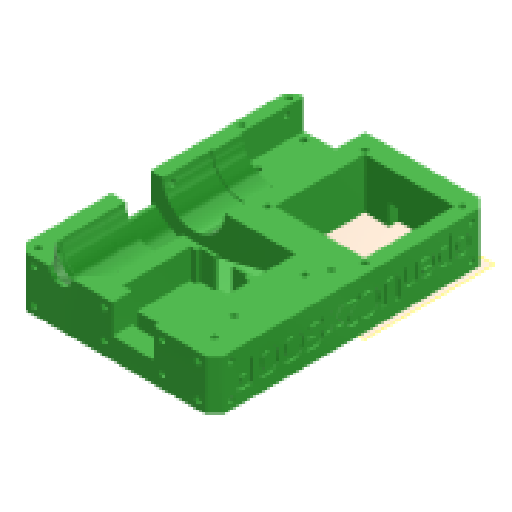
# Autodesk Inventor part: 60_Planktoscope_Base_half1
Saved by Autodesk Inventor 2024.1 (Build 281209000, 209)
## iProperties
Created: 2024-03-03
Part Number: 60_Planktoscope_Base_half1
Material: Generisch
Document SubType Name: Modeling
Designer: diederichbenedict
Density: 1 g/cm^3
Appearance: Glatt - Waldgrün
Author: diederichbenedict
Autodesk Inventor part; units mm, degrees
(part 1 of 2)
ref_plane "YZ Plane" through (0, 0, 0) normal (1, 0, 0) x (0, 1, 0)
ref_plane "XZ Plane" through (0, 0, 0) normal (0, 1, 0) x (-1, 0, 0)
ref_plane "XY Plane" through (0, 0, 0) normal (0, 0, 1) x (1, 0, 0)
ref_plane "Arbeitsebene1" through (0, 0, 0) normal (0, 0, 1) x (1, 0, 0)
ref_plane "Arbeitsebene2" through (-59.4, -108.46, 24.3) normal (0, 0, -1) x (0, 1, 0)
sketch "Skizze1" plane through (0, 0, 0) normal (0, 0, 1) x (1, 0, 0)
  line L0 (-24.5, 28.5) -> (24.5, 28.5) construction
  arc A0 (-24.5, 28.5) -> (-28.5, 24.5) centre (-24.5, 24.5) ccw construction
  line L1 (-28.5, -24.5) -> (-28.5, 24.5) construction
  arc A1 (-28.5, -24.5) -> (-24.5, -28.5) centre (-24.5, -24.5) ccw construction
  line L2 (24.5, -28.5) -> (-24.5, -28.5) construction
  arc A2 (24.5, -28.5) -> (28.5, -24.5) centre (24.5, -24.5) ccw construction
  line L3 (28.5, 24.5) -> (28.5, -24.5) construction
  arc A3 (28.5, 24.5) -> (24.5, 28.5) centre (24.5, 24.5) ccw construction
  circle A4 centre (15.5, -15.5) radius 2 construction
  circle A5 centre (-15.5, -15.5) radius 2 construction
  circle A6 centre (-15.5, 15.5) radius 2 construction
  circle A7 centre (15.5, 15.5) radius 2 construction
  circle A8 centre (0, 0) radius 11.5 construction
  circle A9 centre (23.5, -23.5) radius 2 construction
  circle A10 centre (-23.5, -23.5) radius 2 construction
  circle A11 centre (-23.5, 23.5) radius 2 construction
  circle A12 centre (23.5, 23.5) radius 2 construction
  line L4 (21.15, 14.15) -> (21.15, -14.15) construction
  line L5 (14.15, 21.15) -> (21.15, 14.15) construction
  line L6 (-14.15, 21.15) -> (14.15, 21.15) construction
  line L7 (-21.15, 14.15) -> (-14.15, 21.15) construction
  line L8 (-21.15, -14.15) -> (-21.15, 14.15) construction
  line L9 (-14.15, -21.15) -> (-21.15, -14.15) construction
  line L10 (14.15, -21.15) -> (-14.15, -21.15) construction
  line L11 (21.15, -14.15) -> (14.15, -21.15) construction
  line L12 (17.15, 21.15) -> (14.15, 21.15) construction
  line L13 (21.15, 14.15) -> (14.15, 21.15) construction
  line L14 (21.15, 14.15) -> (21.15, 17.15) construction
  line L15 (21.15, 17.15) -> (17.15, 21.15) construction
  line L16 (21.1433, 21.15) -> (-21.15, 21.15) construction
  line L17 (-21.15, 21.15) -> (-21.15, -21.15) construction
  line L18 (-21.15, -21.15) -> (21.1433, -21.15) construction
  line L19 (21.1433, -21.15) -> (21.1433, 21.15) construction
  line L20 (21.6433, 21.65) -> (-21.65, 21.65)
  line L21 (-21.65, 21.65) -> (-21.65, -21.65)
  line L22 (-21.65, -21.65) -> (21.6433, -21.65)
  line L23 (21.6433, -21.65) -> (21.6433, 21.65)
  circle A13 centre (23.5, 23.5) radius 1.4
  circle A14 centre (23.5, -23.5) radius 1.4
  circle A15 centre (-23.5, 23.5) radius 1.4
  circle A16 centre (-23.5, -23.5) radius 1.4
  line L24 (-58.0629, 31.15) -> (-46.7147, 31.15) construction
  line L25 (-24.5, 28.5) -> (24.5, 28.5) construction
  line L26 (-58.15, -108.944) -> (-33.15, -108.944) construction
  line L27 (-60.15, 4.6456) -> (-60.15, 29.65) construction
  line L28 (28.5, 31.15) -> (-66.5, 31.15) construction
  line L29 (-66.5, 31.15) -> (-66.5, -100.85) construction
  line L30 (-66.5, -100.85) -> (28.5, -100.85) construction
  line L31 (28.5, -100.85) -> (28.5, 31.15) construction
  line L32 (28.5, 31.15) -> (-66.5, 31.15)
  line L33 (-66.5, 31.15) -> (-66.5, -100.85)
  line L34 (-66.5, -100.85) -> (28.5, -100.85)
  line L35 (28.5, -100.85) -> (28.5, 31.15)
  circle A17 centre (-34.65, 27.15) radius 1.6 projected
  circle A18 centre (-35.65, 4.15) radius 1.55 projected
  arc A19 (-35.0696, 29.65) -> (-37.5716, 27.1718) centre (-35.0717, 27.15) ccw construction
  line L36 (-32.3578, 29.6503) -> (-35.0696, 29.6501) construction
  line L37 (-32.3578, 29.6503) -> (-32.3574, 2.149) construction
  spline S0 degree 3 poles (-33.2494, 1.4648) (-33.1945, 1.4704) (-33.1402, 1.4798) (-33.0852, 1.4932) (-33.0302, 1.5066) (-32.9745, 1.5241) (-32.9218, 1.5443) (-32.869, 1.5646) (-32.8192, 1.5877) (-32.7741, 1.6117) (-32.729, 1.6358) (-32.6887, 1.6608) (-32.6523, 1.6864) (-32.6158, 1.712) (-32.5833, 1.7382) (-32.5542, 1.7648) (-32.5251, 1.7914) (-32.4996, 1.8183) (-32.4775, 1.8453) (-32.4554, 1.8722) (-32.4367, 1.899) (-32.4213, 1.9255) (-32.4059, 1.952) (-32.3937, 1.978) (-32.3842, 2.0033) (-32.3747, 2.0286) (-32.3679, 2.0532) (-32.3636, 2.0778) (-32.3593, 2.1023) (-32.3574, 2.1268) (-32.3574, 2.149) knots 0 0 0 0 0.1 0.1 0.1 0.2 0.2 0.2 0.3 0.3 0.3 0.4 0.4 0.4 0.5 0.5 0.5 0.6 0.6 0.6 0.7 0.7 0.7 0.8 0.8 0.8 0.9 0.9 0.9 1 1 1 1 construction
  spline S1 degree 3 poles (-58.0506, 1.4648) (-57.9483, 1.4544) (-57.7309, 1.4485) (-57.3891, 1.4505) (-57.0142, 1.4499) (-56.6055, 1.45) (-56.1597, 1.45) (-55.6728, 1.45) (-55.1399, 1.45) (-54.5557, 1.45) (-53.9136, 1.45) (-53.2059, 1.45) (-52.4235, 1.45) (-51.5547, 1.45) (-50.5859, 1.45) (-49.498, 1.45) (-48.2725, 1.45) (-46.9373, 1.45) (-45.5731, 1.45) (-44.2623, 1.45) (-43.0442, 1.45) (-41.9119, 1.45) (-40.8595, 1.45) (-39.8813, 1.45) (-38.9722, 1.45) (-38.1274, 1.45) (-37.3425, 1.45) (-36.6135, 1.45) (-35.9369, 1.45) (-35.3097, 1.45) (-34.7295, 1.45) (-34.1949, 1.45) (-33.7068, 1.4499) (-33.3956, 1.4501) (-33.2494, 1.4648) knots 0 0 0 0 0.012454 0.026265 0.041356 0.057789 0.075708 0.095278 0.116688 0.140158 0.165945 0.194355 0.225757 0.26059 0.299437 0.342945 0.392182 0.44767 0.504448 0.55719 0.606219 0.651791 0.694148 0.733518 0.770107 0.804111 0.835704 0.865049 0.892289 0.917546 0.940917 0.962464 0.982201 1 1 1 1 construction
  spline S2 degree 3 poles (-58.9429, 2.1479) (-58.9428, 2.1323) (-58.9408, 2.1003) (-58.9319, 2.0518) (-58.9165, 2.0024) (-58.8947, 1.9528) (-58.866, 1.9029) (-58.8299, 1.8528) (-58.786, 1.8026) (-58.7333, 1.7522) (-58.6711, 1.7019) (-58.5978, 1.6519) (-58.512, 1.6028) (-58.4118, 1.556) (-58.2981, 1.5143) (-58.1761, 1.4822) (-58.092, 1.469) (-58.0506, 1.4648) knots 0.000644 0.000644 0.000644 0.000644 0.046478 0.094952 0.144249 0.194804 0.247064 0.301535 0.358802 0.419552 0.484614 0.554981 0.631878 0.716385 0.809647 0.906987 1 1 1 1 construction
  line L38 (-58.9426, 2.1485) -> (-58.9422, 29.6503) construction
  line L39 (-58.9422, 29.6503) -> (-56.2298, 29.6501) construction
  arc A20 (-53.7284, 27.1718) -> (-56.2298, 29.65) centre (-56.2283, 27.15) ccw construction
  line L40 (-53.7228, 26.5387) -> (-53.7284, 27.1718) construction
  arc A21 (-53.7228, 26.5387) -> (-52.4229, 25.25) centre (-52.4229, 26.55) ccw construction
  line L41 (-38.8771, 25.25) -> (-52.4229, 25.25) construction
  arc A22 (-38.8771, 25.25) -> (-37.5772, 26.5387) centre (-38.8771, 26.55) ccw construction
  line L42 (-37.5772, 26.5387) -> (-37.5716, 27.1718) construction
  circle A23 centre (-56.65, 27.15) radius 1.6 projected
  line L43 (-58.35, 24.2) -> (-35.55, 24.2) construction
  line L44 (-58.35, 8.8) -> (-58.35, 24.2) construction
  line L45 (-32.95, 8.8) -> (-58.35, 8.8) construction
  line L46 (-32.95, 21.2) -> (-32.95, 8.8) construction
  line L47 (-35.55, 24.2) -> (-32.95, 21.2) construction
  circle A24 centre (-55.65, 4.15) radius 1.55 projected
  circle A25 centre (-51.65, 5.65) radius 1.1 construction
  circle A26 centre (-39.65, 5.65) radius 1.1 construction
  circle A27 centre (-35.65, 4.15) radius 1.55 construction
  circle A28 centre (-34.65, 27.15) radius 1.6 construction
  point P0 (0, 0)
  dimension "d0" = 0.5
  dimension "d1" = 2.8
  dimension "d2" = 2.8
  dimension "d3" = 2.8
  dimension "d4" = 2.8
  dimension "d5" = 95
  dimension "d6" = 132
  dimension "d41" = 31.15
  constraints: 32 end point, 8 parallel, 4 centre point, 4 coincident, 4 perpendicular, 3 horizontal, 3 other
  measures "d0" distance between parallel lines of L19 L23
  measures "d1" diameter of A13
  measures "d2" diameter of A14
  measures "d3" diameter of A15
  measures "d4" diameter of A16
  measures "d5" distance of L30.end L29.end
  measures "d6" distance of L29.end L28.end
  measures "d41" distance from line of L28 point (0, 0)
extrude "Extrusion1" add sketch "Skizze1" along normal up to surface (24.3 mm away)
sketch "Skizze2" plane through (-66.5, 31.15, 24.3) normal (0, 0, 1) x (1, 0, 0)
  line L0 (44.85, -9.5) -> (88.1433, -9.5) projected
  line L1 (88.1433, -9.5) -> (88.1433, -52.8) projected
  line L2 (88.1433, -52.8) -> (44.85, -52.8) projected
  line L3 (44.85, -52.8) -> (44.85, -9.5) projected
  circle A0 centre (90, -7.65) radius 1.4 projected
  circle A1 centre (90, -54.65) radius 1.4 projected
  circle A2 centre (43, -7.65) radius 1.4 projected
  circle A3 centre (43, -54.65) radius 1.4 projected
  circle A4 centre (31.85, -4) radius 1.6 projected
  circle A5 centre (30.85, -27) radius 1.55 projected
  circle A6 centre (9.85, -4) radius 1.6 projected
  circle A7 centre (10.85, -27) radius 1.55 projected
  line L4 (95, 0) -> (0, 0) projected
  line L5 (0, 0) -> (0, -132) projected
  line L6 (0, -132) -> (95, -132) projected
  line L7 (95, -132) -> (95, 0) projected
  line L8 (7.35, -118.91) -> (7.35, -120.06)
  arc A8 (7.35, -118.91) -> (7.35, -117.91) centre (7.35, -118.41) ccw construction
  line L9 (7.35, -96.06) -> (7.35, -117.91) construction
  line L10 (7.35, -85.56) -> (7.35, -94.56)
  line L11 (6.25, -85.56) -> (35.45, -85.56) projected
  line L12 (6.25, -70.56) -> (6.25, -85.56)
  line L13 (6.25, -44.56) -> (6.25, -70.06)
  line L14 (6.9535, -41.86) -> (6.8517, -30.1979)
  line L15 (33.2, -30.2) -> (33.2, -41.66)
  line L16 (6.9, -41.86) -> (6.9, -44.56)
  line L17 (6.25, -44.56) -> (35.45, -44.56) projected
  line L18 (20.85, -132) -> (20.85, 0) construction
  line L19 (15.35, -128.06) -> (15.35, -132)
  line L20 (7.35, -96.06) -> (7.35, -94.56)
  line L21 (7.35, -85.56) -> (6.25, -85.56)
  line L22 (6.25, -70.56) -> (6.25, -70.06)
  line L23 (15.1, -132) -> (15.1, -128.1636)
  line L24 (7.1, -120.1636) -> (7.1, -118.41)
  arc A9 (7.1, -118.41) -> (7.1, -118.41) centre (7.35, -118.41) ccw
  line L25 (7.1, -118.41) -> (7.1, -96.0507)
  line L26 (7.1, -96.0507) -> (7.1, -94.56)
  line L27 (7.1, -94.56) -> (7.1, -85.81)
  line L28 (7.1, -85.81) -> (6, -85.81)
  line L29 (6, -85.81) -> (6, -70.56)
  line L30 (6, -70.56) -> (6, -70.06)
  line L31 (6, -70.06) -> (6, -44.31)
  line L32 (6, -44.31) -> (35.45, -44.31)
  line L33 (6.8, -44.31) -> (6.8, -30.064)
  line L34 (6.8, -30.064) -> (20.85, -30.064)
  line L35 (20.85, -30.064) -> (20.85, -132)
  line L36 (15.1, -132) -> (20.85, -132)
  line L37 (7.1, -97.4127) -> (7.2407, -96.0654)
  line L38 (7.2407, -96.0654) -> (7.1, -96.0507)
  circle A10 centre (7.1, -117.9136) radius 0.5
  line L39 (7.35, -120.06) -> (15.35, -129.594) construction
  line L40 (15.35, -130.03) -> (7.1, -120.198)
  line L41 (7.1, -120.198) -> (7.1, -120.1636)
  point P0 (66.5, -31.15)
  point P1 (20.85, -85.56)
  point P2 (20.85, -44.56)
  point P3 (20.85, -44.31)
  point P4 (7.1, -118.4136)
  point P5 (7.1, -117.4136)
  point P6 (15.1, -129.7321)
  point P7 (6.9, -44.31)
  dimension "d9" = 0.25
  dimension "d74" = 1
  dimension "d75" = 2.25
  constraints: 64 end point, 11 vertical, 7 point on line, 5 perpendicular, 4 point on circle, 3 centre point, 2 collinear, 1 horizontal, 1 midpoint, 1 parallel, 30 other
  measures "d9" distance between parallel lines of L9 L25
  measures "d74" diameter of A10
  measures "d75" distance of A10.centre L24.start
revolve "Umdrehung1" cut sketch "Skizze2" angle 360 about axis through (-45.65, -100.85, 24.3) along (0, 1, 0) contours L6 L19 L40 L41 L24 A9 A10 L25 L37 L38 L26 L27 L28 L29 L30 L31 L32 L16 L17 L13 L22 L12 L11 L35 | L11 L12 L22 L13 L17 L35 | L17 L16 L32 L35 | L32 L33 L34 L35 | A10 A9
sketch "Skizze3" plane through (-66.5, 31.15, 24.3) normal (0, 0, 1) x (1, 0, 0)
  line L0 (41.8499, -119.66) -> (41.8499, -113.96) projected
  line L1 (69.8499, -119.66) -> (69.8499, -113.96) projected
  line L2 (47.9499, -122.06) -> (63.7499, -122.06) projected
  line L3 (44.8499, -88.76) -> (66.8499, -88.76) projected
  line L4 (44.8499, -90.56) -> (44.8499, -88.76)
  line L5 (66.8499, -90.56) -> (66.8499, -88.76)
  line L6 (41.8499, -122.06) -> (69.8499, -122.06)
  line L7 (69.8499, -122.06) -> (69.8499, -90.56)
  line L8 (69.8499, -90.56) -> (41.8499, -90.56)
  line L9 (41.8499, -90.56) -> (41.8499, -122.06)
  line L10 (65.8499, -140.6578) -> (45.8499, -140.6578)
  line L11 (45.8499, -140.6578) -> (45.8499, -122.06)
  line L12 (45.8499, -122.06) -> (65.8499, -122.06)
  line L13 (65.8499, -122.06) -> (65.8499, -140.6578)
  line L14 (65.8499, -140.6578) -> (45.8499, -122.06) construction
  line L15 (45.8499, -140.6578) -> (65.8499, -122.06) construction
  line L16 (41.3499, -122.56) -> (70.3499, -122.56)
  line L17 (70.3499, -122.56) -> (70.3499, -90.06)
  line L18 (70.3499, -90.06) -> (41.3499, -90.06)
  line L19 (41.3499, -90.06) -> (41.3499, -122.56)
  line L20 (67.3499, -90.56) -> (67.3499, -88.26)
  line L21 (67.3499, -88.26) -> (44.3499, -88.26)
  line L22 (44.3499, -88.26) -> (44.3499, -90.56)
  line L23 (60.0306, -74.6503) -> (51.6692, -74.6503)
  line L24 (51.6692, -74.6503) -> (51.6692, -88.26)
  line L25 (51.6692, -88.26) -> (60.0306, -88.26)
  line L26 (60.0306, -88.26) -> (60.0306, -74.6503)
  line L27 (60.0306, -74.6503) -> (51.6692, -88.26) construction
  line L28 (51.6692, -74.6503) -> (60.0306, -88.26) construction
  point P0 (66.5, -31.15)
  point P1 (55.8499, -131.3589)
  point P2 (55.8499, -81.4552)
  point P3 (44.3499, -90.06)
  point P4 (45.8499, -122.56)
  point P5 (65.8499, -122.56)
  point P6 (67.3499, -90.06)
  dimension "d11" = 20
  dimension "d12" = 0.5
  dimension "d13" = 0.5
  constraints: 50 end point, 8 parallel, 4 midpoint, 4 perpendicular, 3 horizontal, 2 point on line, 2 vertical, 7 other
  measures "d11" distance of L11.end L12.end
  measures "d12" distance between parallel lines of L9 L19
  measures "d13" distance between parallel lines of L3 L21
extrude "Extrusion2" cut sketch "Skizze3" against normal blind 14.1
sketch "Skizze4" plane through (-60.5, -54.66, 24.3) normal (0, 1, 0) x (1, 0, 0)
  arc A0 (14.7163, 14.1976) -> (0.6736, 0.7871) centre (14.85, 0) ccw projected
  circle A1 centre (49.8499, -0.1) radius 2.3 projected
  circle A2 centre (14.85, 0) radius 14.1983
  circle A3 centre (49.8499, -0.1) radius 6
  circle A4 centre (14.85, 0) radius 22.1983
  circle A5 centre (49.8499, -0.1) radius 14
  line L0 (20.1113, 21.5658) -> (53.168, 13.5011)
  line L1 (49.8499, -0.1) -> (14.85, 0)
  point P0 (60.5, 24.3)
  point P1 (37.0482, -0.0634)
  point P2 (35.8499, -0.06)
  point P3 (36.5766, -4.5519)
  point P4 (36.6022, 4.4277)
  dimension "d16" = 12
  dimension "d17" = 8
  dimension "d18" = 8
  constraints: 4 end point, 2 centre point, 2 coincident, 1 concentric, 8 other
  measures "d16" diameter of A3
extrude "Extrusion3" cut sketch "Skizze4" along normal blind 18 and the other way blind 1 contours A2 A0 | A1 | A3 | A4 L1 A5 | A4 A5 | A5 A4 | A4 L0 A5 | A4 A5 L1
sketch "Skizze5" plane through (-66.5, 31.15, 24.3) normal (0, 0, 1) x (1, 0, 0)
  line L0 (60.0306, -86.81) -> (60.0306, -88.26) projected
  line L1 (60.0306, -88.26) -> (67.3499, -88.26) projected
  line L2 (67.3499, -88.26) -> (67.3499, -90.06) projected
  line L3 (67.3499, -90.06) -> (70.3499, -90.06) projected
  line L4 (70.3499, -90.06) -> (70.3499, -122.56) projected
  line L5 (70.3499, -122.56) -> (65.8499, -122.56) projected
  line L6 (65.8499, -122.56) -> (65.8499, -132) projected
  line L7 (65.8499, -132) -> (95, -132) projected
  line L8 (95, -132) -> (95, 0) projected
  line L9 (95, 0) -> (0, 0) projected
  line L10 (26.35, -132) -> (45.8499, -132) projected
  line L11 (44.85, -9.5) -> (88.1433, -9.5) projected
  line L12 (88.1433, -9.5) -> (88.1433, -52.8) projected
  line L13 (88.1433, -52.8) -> (44.85, -52.8) projected
  line L14 (44.85, -52.8) -> (44.85, -9.5) projected
  circle A0 centre (90, -7.65) radius 1.4 projected
  circle A1 centre (90, -54.65) radius 1.4 projected
  circle A2 centre (43, -7.65) radius 1.4 projected
  circle A3 centre (43, -54.65) radius 1.4 projected
  circle A4 centre (31.85, -4) radius 1.6 projected
  circle A5 centre (30.85, -27) radius 1.55 projected
  circle A6 centre (9.85, -4) radius 1.6 projected
  circle A7 centre (10.85, -27) radius 1.55 projected
  line L15 (35.35, -1.5) -> (35.35, -27) projected
  line L16 (6.35, -26.9997) -> (6.35, -1.5) projected
  line L17 (35.35, -30.064) -> (6.35, -30.064)
  line L18 (6.35, -30.064) -> (6.35, 0)
  line L19 (6.35, 0) -> (35.35, 0)
  line L20 (35.35, 0) -> (35.35, -30.064)
  line L21 (35.65, -30.364) -> (6.05, -30.364)
  line L22 (6.05, -30.364) -> (6.05, 0.3)
  line L23 (6.05, 0.3) -> (35.65, 0.3)
  line L24 (35.65, 0.3) -> (35.65, -30.364)
  line L25 (45.8499, -132) -> (45.8499, -122.56) projected
  line L26 (45.8499, -122.56) -> (41.3499, -122.56) projected
  line L27 (41.3499, -122.56) -> (41.3499, -90.06) projected
  line L28 (41.3499, -90.06) -> (44.3499, -90.06) projected
  line L29 (44.3499, -90.06) -> (44.3499, -88.26) projected
  line L30 (44.3499, -88.26) -> (51.6692, -88.26) projected
  line L31 (51.6692, -88.26) -> (51.6692, -86.81) projected
  line L32 (0, -86.81) -> (0, -132) projected
  line L33 (51.6692, -86.81) -> (34.6, -86.81) projected
  line L34 (34.6, -86.81) -> (34.6, -96.0507) projected
  line L35 (34.6, -96.0507) -> (34.4593, -96.0654) projected
  line L36 (34.4593, -96.0654) -> (34.6, -97.4127) projected
  line L37 (34.6, -97.4127) -> (34.6, -117.4136) projected
  arc A8 (34.6, -117.4136) -> (34.6, -118.4136) centre (34.6, -117.9136) ccw projected
  line L38 (34.6, -118.4136) -> (34.6, -120.198) projected
  line L39 (34.6, -120.198) -> (26.35, -130.03) projected
  line L40 (26.35, -130.03) -> (26.35, -132) projected
  line L41 (69.8495, -86.81) -> (60.0306, -86.81) projected
  line L42 (0, 0) -> (0, -67.81) projected
  line L43 (0, -67.81) -> (6, -67.81) projected
  line L44 (6, -67.81) -> (6, -44.31) projected
  line L45 (6, -44.31) -> (6.8, -44.31) projected
  line L46 (6.8, -44.31) -> (6.8, -30.064) projected
  line L47 (6.8, -30.064) -> (34.9, -30.064) projected
  line L48 (34.9, -30.064) -> (34.9, -44.31) projected
  line L49 (34.9, -44.31) -> (35.7, -44.31) projected
  line L50 (35.7, -44.31) -> (35.7, -67.81) projected
  line L51 (35.7, -67.81) -> (69.8495, -67.81) projected
  line L52 (69.8495, -67.81) -> (69.8495, -86.81) projected
  line L53 (7.1, -86.81) -> (0, -86.81) projected
  line L54 (0, -132) -> (15.35, -132) projected
  line L55 (15.35, -132) -> (15.35, -130.03) projected
  line L56 (15.35, -130.03) -> (7.1, -120.198) projected
  line L57 (7.1, -120.198) -> (7.1, -118.4136) projected
  arc A9 (7.1, -118.4136) -> (7.1, -117.4136) centre (7.1, -117.9136) ccw projected
  line L58 (7.1, -117.4136) -> (7.1, -97.4127) projected
  line L59 (7.1, -97.4127) -> (7.2407, -96.0654) projected
  line L60 (7.2407, -96.0654) -> (7.1, -96.0507) projected
  line L61 (7.1, -96.0507) -> (7.1, -86.81) projected
  point P0 (66.5, -31.15)
  dimension "d23" = 0.3
  constraints: 16 end point, 4 parallel, 2 perpendicular, 1 horizontal, 1 point on line, 3 other
  measures "d23" distance between parallel lines of L20 L24
extrude "Extrusion4" cut sketch "Skizze5" against normal blind 14.3 contours L48 L17 L20 L15 L9 L24 L21 | L21 L46 L17 L48 | L21 L22 L9 L18 L16 L17 L46 | L17 L18 L16 L9 L20 L15 | L9 L22 L23 L24 | A4 | A5 | A6 | A7
sketch "Skizze6" plane through (0, 0, 0) normal (0, 0, -1) x (-1, 0, 0)
  line L0 (66.5, 31.15) -> (66.5, -100.85) construction
  line L1 (-28.5, 31.15) -> (66.5, 31.15) construction
  line L2 (-28.5, -100.85) -> (-28.5, 31.15) construction
  line L3 (66.5, -100.85) -> (-28.5, -100.85) construction
  circle A0 centre (55.65, 4.15) radius 1.55 projected
  circle A1 centre (56.65, 27.15) radius 1.6 projected
  circle A2 centre (35.65, 4.15) radius 1.55 projected
  circle A3 centre (34.65, 27.15) radius 1.6 projected
  circle A4 centre (23.5, -23.5) radius 1.4 projected
  circle A5 centre (23.5, 23.5) radius 1.4 projected
  circle A6 centre (-23.5, -23.5) radius 1.4 projected
  circle A7 centre (-23.5, 23.5) radius 1.4 projected
  line L4 (-21.6433, 21.65) -> (-21.6433, -21.65) projected
  line L5 (21.65, 21.65) -> (-21.6433, 21.65) projected
  line L6 (21.65, -21.65) -> (21.65, 21.65) projected
  line L7 (-21.6433, -21.65) -> (21.65, -21.65) projected
  line L8 (-18.5, -90.85) -> (-18.5, 21.15) construction
  line L9 (-18.5, 21.15) -> (56.5, 21.15) construction
  line L10 (56.5, 21.15) -> (56.5, -90.85) construction
  line L11 (56.5, -90.85) -> (-18.5, -90.85) construction
  point P0 (0, 0)
  point P1 (-18.5, -34.85)
  point P2 (-14.0855, -43.0199)
  point P3 (-14.0855, -77.1359)
  point P4 (63.5, 27.15)
  point P5 (63.5, 4.15)
  point P6 (61.2633, -96.1146)
  dimension "d26" = 10
  dimension "d34" = 3
  dimension "d35" = 3
  constraints: 8 end point, 2 coincident, 1 midpoint, 3 other
  measures "d26" distance between parallel lines of L3 L11
  measures "d34" distance from line of point (63.5, 4.15) L0
  measures "d35" distance from line of L0 point (63.5, 27.15)
hole "Bohrung1" at (18.5, -90.85, 0) at (18.5, -34.85, 0) at (14.0855, -43.0199, 0) at (14.0855, -77.1359, 0) at (-63.5, 4.15, 0) at (-63.5, 27.15, 0) at (-61.2633, -96.1146, 0) direction (0, 0, 1) diameter 2.8 end through all counterbore diameter 6.5 counterbore depth 8
chamfer "Fasen1" distance 4 angle 45 4 edges at (-66.5, -100.85, 12.15) (-66.5, 31.15, 12.15) (28.5, -100.85, 12.15) (28.5, 31.15, 12.15)
sketch "Skizze7" plane through (28.5, -96.85, 0) normal (1, 0, 0) x (0, 0, -1)
  line L0 (-5.6102, 119.9159) -> (-5.6102, 5.5404) construction
  line L1 (-5.6102, 5.5404) -> (-2.1331, 5.5404) construction
  line L2 (-2.1331, 5.5404) -> (-2.1331, 119.9159) construction
  line L3 (-2.1331, 119.9159) -> (-5.6102, 119.9159) construction
  spline S0 degree 2 poles (-12.853, 111.9734) (-14.9795, 111.9734) (-17.2968, 114.0181) (-17.2968, 115.7266) knots 0 0 0 1 2 2 2
  spline S1 degree 2 poles (-17.2968, 115.7266) (-17.2968, 117.4805) (-14.9068, 119.4888) (-12.853, 119.4888) knots 0 0 0 1 2 2 2
  spline S2 degree 2 poles (-12.853, 119.4888) (-10.7447, 119.4888) (-8.4092, 117.4168) (-8.4092, 115.7266) knots 0 0 0 1 2 2 2
  spline S3 degree 2 poles (-8.4092, 115.7266) (-8.4092, 114.0181) (-10.7356, 111.9734) (-12.853, 111.9734) knots 0 0 0 1 2 2 2
  spline S4 degree 2 poles (-12.853, 113.4365) (-11.2172, 113.4365) (-9.6269, 114.627) (-9.6269, 115.7266) knots 0 0 0 1 2 2 2
  spline S5 degree 2 poles (-9.6269, 115.7266) (-9.6269, 116.8262) (-11.2172, 118.0257) (-12.853, 118.0257) knots 0 0 0 1 2 2 2
  spline S6 degree 2 poles (-12.853, 118.0257) (-14.4433, 118.0257) (-16.0791, 116.8262) (-16.0791, 115.7266) knots 0 0 0 1 2 2 2
  spline S7 degree 2 poles (-16.0791, 115.7266) (-16.0791, 114.6361) (-14.4706, 113.4365) (-12.853, 113.4365) knots 0 0 0 1 2 2 2
  spline S8 degree 2 poles (-12.6258, 103.4675) (-14.7341, 103.4675) (-17.2241, 105.4758) (-17.2241, 107.0116) knots 0 0 0 1 2 2 2
  spline S9 degree 2 poles (-17.2241, 107.0116) (-17.2241, 107.6387) (-16.9333, 108.6019) (-16.6334, 109.1018) knots 0 0 0 1 2 2 2
  line L4 (-16.6334, 109.1018) -> (-20.1594, 109.1018)
  line L5 (-20.1594, 109.1018) -> (-20.1594, 110.5194)
  line L6 (-20.1594, 110.5194) -> (-8.6455, 110.5194)
  line L7 (-8.6455, 110.5194) -> (-8.6455, 109.1018)
  line L8 (-8.6455, 109.1018) -> (-9.527, 109.1018)
  spline S10 degree 2 poles (-9.527, 109.1018) (-9.0453, 108.5747) (-8.4092, 107.2843) (-8.4092, 106.53) knots 0 0 0 1 2 2 2
  spline S11 degree 2 poles (-8.4092, 106.53) (-8.4092, 105.0851) (-10.6992, 103.4675) (-12.6258, 103.4675) knots 0 0 0 1 2 2 2
  spline S12 degree 2 poles (-12.7894, 104.9306) (-11.3445, 104.9306) (-9.7541, 105.8484) (-9.7541, 106.8753) knots 0 0 0 1 2 2 2
  spline S13 degree 2 poles (-9.7541, 106.8753) (-9.7541, 107.4751) (-10.2903, 108.6019) (-10.7083, 109.1018) knots 0 0 0 1 2 2 2
  line L9 (-10.7083, 109.1018) -> (-15.4884, 109.1018)
  spline S14 degree 2 poles (-15.4884, 109.1018) (-15.7519, 108.5474) (-15.9518, 107.7568) (-15.9518, 107.2479) knots 0 0 0 1 2 2 2
  spline S15 degree 2 poles (-15.9518, 107.2479) (-15.9518, 106.1483) (-14.3343, 104.9306) (-12.7894, 104.9306) knots 0 0 0 1 2 2 2
  spline S16 degree 2 poles (-17.2513, 98.3421) (-17.2513, 100.3596) (-14.9886, 102.5769) (-12.8984, 102.5769) knots 0 0 0 1 2 2 2
  spline S17 degree 2 poles (-12.8984, 102.5769) (-10.8446, 102.5769) (-8.4092, 100.4232) (-8.4092, 98.6875) knots 0 0 0 1 2 2 2
  spline S18 degree 2 poles (-8.4092, 98.6875) (-8.4092, 97.9059) (-8.8636, 96.6973) (-9.3452, 96.252) knots 0 0 0 1 2 2 2
  spline S19 degree 2 poles (-9.3452, 96.252) (-9.8268, 95.7976) (-11.2172, 95.316) (-12.2259, 95.316) knots 0 0 0 1 2 2 2
  line L10 (-12.2259, 95.316) -> (-12.9984, 95.316)
  line L11 (-12.9984, 95.316) -> (-12.9984, 101.1411)
  spline S20 degree 2 poles (-12.9984, 101.1411) (-14.4615, 101.1411) (-16.0154, 99.6689) (-16.0154, 98.3603) knots 0 0 0 1 2 2 2
  spline S21 degree 2 poles (-16.0154, 98.3603) (-16.0154, 97.8968) (-15.8064, 96.9972) (-15.6429, 96.6337) knots 0 0 0 1 2 2 2
  spline S22 degree 2 poles (-15.6429, 96.6337) (-15.4611, 96.252) (-15.143, 95.7249) (-14.9976, 95.5523) knots 0 0 0 1 2 2 2
  line L12 (-14.9976, 95.5523) -> (-14.9976, 95.4705)
  line L13 (-14.9976, 95.4705) -> (-16.5425, 95.4705)
  spline S23 degree 2 poles (-16.5425, 95.4705) (-16.6425, 95.7158) (-16.9333, 96.461) (-17.0151, 96.7518) knots 0 0 0 1 2 2 2
  spline S24 degree 2 poles (-17.0151, 96.7518) (-17.1332, 97.1608) (-17.2513, 97.8332) (-17.2513, 98.3421) knots 0 0 0 1 2 2 2
  spline S25 degree 2 poles (-11.917, 96.6973) (-11.3445, 96.7155) (-10.5084, 96.9517) (-10.2267, 97.1789) knots 0 0 0 1 2 2 2
  spline S26 degree 2 poles (-10.2267, 97.1789) (-9.9086, 97.4243) (-9.5724, 98.1967) (-9.5724, 98.7692) knots 0 0 0 1 2 2 2
  spline S27 degree 2 poles (-9.5724, 98.7692) (-9.5724, 99.3327) (-9.9086, 100.1233) (-10.2358, 100.4504) knots 0 0 0 1 2 2 2
  spline S28 degree 2 poles (-10.2358, 100.4504) (-10.572, 100.7685) (-11.3808, 101.0957) (-11.917, 101.1411) knots 0 0 0 1 2 2 2
  line L14 (-11.917, 101.1411) -> (-11.917, 96.6973)
  line L15 (-17.0605, 87.2735) -> (-17.0605, 88.6912)
  line L16 (-17.0605, 88.6912) -> (-12.2623, 88.6912)
  spline S29 degree 2 poles (-12.2623, 88.6912) (-11.6807, 88.6912) (-10.6811, 88.8002) (-10.3812, 88.9638) knots 0 0 0 1 2 2 2
  spline S30 degree 2 poles (-10.3812, 88.9638) (-10.0631, 89.1365) (-9.7541, 89.7544) (-9.7541, 90.2815) knots 0 0 0 1 2 2 2
  spline S31 degree 2 poles (-9.7541, 90.2815) (-9.7541, 90.8086) (-10.3176, 91.9263) (-10.7719, 92.4625) knots 0 0 0 1 2 2 2
  line L17 (-10.7719, 92.4625) -> (-17.0605, 92.4625)
  line L18 (-17.0605, 92.4625) -> (-17.0605, 93.8802)
  line L19 (-17.0605, 93.8802) -> (-8.6455, 93.8802)
  line L20 (-8.6455, 93.8802) -> (-8.6455, 92.4625)
  line L21 (-8.6455, 92.4625) -> (-9.5815, 92.4625)
  spline S32 degree 2 poles (-9.5815, 92.4625) (-9.009, 91.8264) (-8.4092, 90.5996) (-8.4092, 89.9089) knots 0 0 0 1 2 2 2
  spline S33 degree 2 poles (-8.4092, 89.9089) (-8.4092, 88.673) (-10.0449, 87.2735) (-11.5989, 87.2735) knots 0 0 0 1 2 2 2
  line L22 (-11.5989, 87.2735) -> (-17.0605, 87.2735)
  spline S34 degree 2 poles (-17.2968, 81.2576) (-17.2968, 82.2481) (-16.7788, 83.7203) (-16.2608, 84.2383) knots 0 0 0 1 2 2 2
  spline S35 degree 2 poles (-16.2608, 84.2383) (-15.6792, 84.829) (-14.0435, 85.3106) (-12.8439, 85.3106) knots 0 0 0 1 2 2 2
  line L23 (-12.8439, 85.3106) -> (-5.8465, 85.3106)
  line L24 (-5.8465, 85.3106) -> (-5.8465, 83.8203)
  line L25 (-5.8465, 83.8203) -> (-12.8439, 83.8203)
  spline S36 degree 2 poles (-12.8439, 83.8203) (-13.6254, 83.8203) (-14.6796, 83.6204) (-15.1067, 83.3386) knots 0 0 0 1 2 2 2
  spline S37 degree 2 poles (-15.1067, 83.3386) (-15.5611, 83.0388) (-16.0245, 82.0028) (-16.0245, 81.2576) knots 0 0 0 1 2 2 2
  spline S38 degree 2 poles (-16.0245, 81.2576) (-16.0245, 80.5579) (-15.5611, 79.4674) (-15.1067, 79.1675) knots 0 0 0 1 2 2 2
  spline S39 degree 2 poles (-15.1067, 79.1675) (-14.6796, 78.8858) (-13.6345, 78.6858) (-12.8802, 78.6858) knots 0 0 0 1 2 2 2
  line L26 (-12.8802, 78.6858) -> (-5.8465, 78.6858)
  line L27 (-5.8465, 78.6858) -> (-5.8465, 77.1955)
  line L28 (-5.8465, 77.1955) -> (-12.8439, 77.1955)
  spline S40 degree 2 poles (-12.8439, 77.1955) (-14.0162, 77.1955) (-15.6883, 77.668) (-16.2608, 78.2678) knots 0 0 0 1 2 2 2
  spline S41 degree 2 poles (-16.2608, 78.2678) (-16.7879, 78.804) (-17.2968, 80.2216) (-17.2968, 81.2576) knots 0 0 0 1 2 2 2
  spline S42 degree 2 poles (-17.2604, 70.6797) (-17.2604, 71.7702) (-16.5243, 73.615) (-15.7883, 74.2875) knots 0 0 0 1 2 2 2
  spline S43 degree 2 poles (-15.7883, 74.2875) (-15.0613, 74.9599) (-12.8802, 75.696) (-11.4626, 75.696) knots 0 0 0 1 2 2 2
  spline S44 degree 2 poles (-11.4626, 75.696) (-10.054, 75.696) (-7.9639, 74.9781) (-7.1915, 74.2966) knots 0 0 0 1 2 2 2
  spline S45 degree 2 poles (-7.1915, 74.2966) (-6.4372, 73.6241) (-5.6466, 71.7884) (-5.6466, 70.6525) knots 0 0 0 1 2 2 2
  spline S46 degree 2 poles (-5.6466, 70.6525) (-5.6466, 70.089) (-5.8102, 69.0985) (-5.9374, 68.6805) knots 0 0 0 1 2 2 2
  spline S47 degree 2 poles (-5.9374, 68.6805) (-6.0555, 68.317) (-6.3918, 67.5627) (-6.5917, 67.1901) knots 0 0 0 1 2 2 2
  line L29 (-6.5917, 67.1901) -> (-8.391, 67.1901)
  line L30 (-8.391, 67.1901) -> (-8.391, 67.3083)
  spline S48 degree 2 poles (-8.391, 67.3083) (-8.2093, 67.5082) (-7.7004, 68.1261) (-7.455, 68.5714) knots 0 0 0 1 2 2 2
  spline S49 degree 2 poles (-7.455, 68.5714) (-7.2187, 68.9985) (-6.9188, 70.0072) (-6.9188, 70.6615) knots 0 0 0 1 2 2 2
  spline S50 degree 2 poles (-6.9188, 70.6615) (-6.9188, 71.3795) (-7.5095, 72.6608) (-8.073, 73.1424) knots 0 0 0 1 2 2 2
  spline S51 degree 2 poles (-8.073, 73.1424) (-8.6455, 73.615) (-10.3812, 74.1421) (-11.4626, 74.1421) knots 0 0 0 1 2 2 2
  spline S52 degree 2 poles (-11.4626, 74.1421) (-12.6167, 74.1421) (-14.2797, 73.5877) (-14.8522, 73.1061) knots 0 0 0 1 2 2 2
  spline S53 degree 2 poles (-14.8522, 73.1061) (-15.4066, 72.6335) (-15.97, 71.3704) (-15.97, 70.6615) knots 0 0 0 1 2 2 2
  spline S54 degree 2 poles (-15.97, 70.6615) (-15.97, 70.0163) (-15.6519, 68.9167) (-15.4157, 68.4896) knots 0 0 0 1 2 2 2
  spline S55 degree 2 poles (-15.4157, 68.4896) (-15.1794, 68.0807) (-14.6887, 67.4718) (-14.516, 67.2992) knots 0 0 0 1 2 2 2
  line L31 (-14.516, 67.2992) -> (-14.516, 67.1901)
  line L32 (-14.516, 67.1901) -> (-16.2972, 67.1901)
  spline S56 degree 2 poles (-16.2972, 67.1901) (-16.4698, 67.5627) (-16.7879, 68.217) (-16.9333, 68.6805) knots 0 0 0 1 2 2 2
  spline S57 degree 2 poles (-16.9333, 68.6805) (-17.0969, 69.1712) (-17.2604, 70.0072) (-17.2604, 70.6797) knots 0 0 0 1 2 2 2
  line L33 (-17.0605, 59.2022) -> (-17.0605, 66.1178)
  line L34 (-17.0605, 66.1178) -> (-15.4702, 66.1178)
  spline S58 degree 2 poles (-15.4702, 66.1178) (-14.7705, 65.3726) (-13.4709, 64.0458) (-12.7712, 63.4097) knots 0 0 0 1 2 2 2
  spline S59 degree 2 poles (-12.7712, 63.4097) (-11.3626, 62.1284) (-9.6724, 61.1924) (-8.7727, 61.1924) knots 0 0 0 1 2 2 2
  spline S60 degree 2 poles (-8.7727, 61.1924) (-8.3001, 61.1924) (-7.5913, 61.4832) (-7.3641, 61.7467) knots 0 0 0 1 2 2 2
  spline S61 degree 2 poles (-7.3641, 61.7467) (-7.1369, 62.0102) (-6.9097, 62.7009) (-6.9097, 63.1189) knots 0 0 0 1 2 2 2
  spline S62 degree 2 poles (-6.9097, 63.1189) (-6.9097, 63.5188) (-7.1097, 64.3366) (-7.2642, 64.7092) knots 0 0 0 1 2 2 2
  spline S63 degree 2 poles (-7.2642, 64.7092) (-7.3914, 65.0273) (-7.7549, 65.618) (-7.8821, 65.7997) knots 0 0 0 1 2 2 2
  line L35 (-7.8821, 65.7997) -> (-7.8821, 65.8815)
  line L36 (-7.8821, 65.8815) -> (-6.2827, 65.8815)
  spline S64 degree 2 poles (-6.2827, 65.8815) (-6.0555, 65.418) (-5.6102, 63.755) (-5.6102, 63.0099) knots 0 0 0 1 2 2 2
  spline S65 degree 2 poles (-5.6102, 63.0099) (-5.6102, 61.4377) (-7.2732, 59.6656) (-8.6909, 59.6656) knots 0 0 0 1 2 2 2
  spline S66 degree 2 poles (-8.6909, 59.6656) (-9.3543, 59.6656) (-10.463, 59.9746) (-10.9355, 60.2472) knots 0 0 0 1 2 2 2
  spline S67 degree 2 poles (-10.9355, 60.2472) (-11.4262, 60.5199) (-12.3895, 61.3105) (-12.853, 61.7467) knots 0 0 0 1 2 2 2
  spline S68 degree 2 poles (-12.853, 61.7467) (-13.6254, 62.4555) (-15.2794, 64.1912) (-15.761, 64.7092) knots 0 0 0 1 2 2 2
  line L37 (-15.761, 64.7092) -> (-15.761, 59.2022)
  line L38 (-15.761, 59.2022) -> (-17.0605, 59.2022)
  line L39 (-17.0605, 49.1696) -> (-17.0605, 52.2593)
  line L40 (-17.0605, 52.2593) -> (-14.6341, 53.8678)
  line L41 (-14.6341, 53.8678) -> (-17.0605, 55.5217)
  line L42 (-17.0605, 55.5217) -> (-17.0605, 58.5479)
  line L43 (-17.0605, 58.5479) -> (-12.8257, 55.4309)
  line L44 (-12.8257, 55.4309) -> (-8.6, 58.4934)
  line L45 (-8.6, 58.4934) -> (-8.6, 55.4036)
  line L46 (-8.6, 55.4036) -> (-10.981, 53.8224)
  line L47 (-10.981, 53.8224) -> (-8.6, 52.2321)
  line L48 (-8.6, 52.2321) -> (-8.6, 49.2059)
  line L49 (-8.6, 49.2059) -> (-12.7621, 52.2684)
  line L50 (-12.7621, 52.2684) -> (-17.0605, 49.1696)
  spline S69 degree 2 poles (-17.2604, 44.5713) (-17.2604, 45.8617) (-16.7606, 47.8064) (-16.3971, 48.6425) knots 0 0 0 1 2 2 2
  line L51 (-16.3971, 48.6425) -> (-13.7254, 48.6425)
  line L52 (-13.7254, 48.6425) -> (-13.7254, 48.388)
  spline S70 degree 2 poles (-13.7254, 48.388) (-14.4433, 47.5429) (-15.2157, 45.5164) (-15.2157, 44.5622) knots 0 0 0 1 2 2 2
  spline S71 degree 2 poles (-15.2157, 44.5622) (-15.2157, 44.3168) (-15.1067, 43.5262) (-14.9976, 43.2899) knots 0 0 0 1 2 2 2
  spline S72 degree 2 poles (-14.9976, 43.2899) (-14.8704, 42.9991) (-14.407, 42.5902) (-14.0344, 42.5902) knots 0 0 0 1 2 2 2
  spline S73 degree 2 poles (-14.0344, 42.5902) (-13.6073, 42.5902) (-13.0802, 43.2536) (-12.962, 43.708) knots 0 0 0 1 2 2 2
  spline S74 degree 2 poles (-12.962, 43.708) (-12.8075, 44.2805) (-12.544, 45.58) (-12.3441, 46.1525) knots 0 0 0 1 2 2 2
  spline S75 degree 2 poles (-12.3441, 46.1525) (-11.8897, 47.452) (-10.3357, 48.5789) (-9.1725, 48.5789) knots 0 0 0 1 2 2 2
  spline S76 degree 2 poles (-9.1725, 48.5789) (-7.6004, 48.5789) (-5.6466, 45.9162) (-5.6466, 43.917) knots 0 0 0 1 2 2 2
  spline S77 degree 2 poles (-5.6466, 43.917) (-5.6466, 42.9173) (-6.0555, 40.9363) (-6.4008, 40.1547) knots 0 0 0 1 2 2 2
  line L53 (-6.4008, 40.1547) -> (-8.9635, 40.1547)
  line L54 (-8.9635, 40.1547) -> (-8.9635, 40.4001)
  spline S78 degree 2 poles (-8.9635, 40.4001) (-8.4274, 41.0271) (-7.6913, 42.8265) (-7.6913, 43.7716) knots 0 0 0 1 2 2 2
  spline S79 degree 2 poles (-7.6913, 43.7716) (-7.6913, 44.1442) (-7.8003, 44.7258) (-7.9457, 45.0529) knots 0 0 0 1 2 2 2
  spline S80 degree 2 poles (-7.9457, 45.0529) (-8.0639, 45.3165) (-8.5364, 45.6981) (-8.8272, 45.6981) knots 0 0 0 1 2 2 2
  spline S81 degree 2 poles (-8.8272, 45.6981) (-9.2634, 45.6981) (-9.7632, 45.0893) (-9.9632, 44.2169) knots 0 0 0 1 2 2 2
  spline S82 degree 2 poles (-9.9632, 44.2169) (-10.0904, 43.6534) (-10.3357, 42.6084) (-10.5448, 42.0086) knots 0 0 0 1 2 2 2
  spline S83 degree 2 poles (-10.5448, 42.0086) (-10.9719, 40.8454) (-12.3895, 39.7095) (-13.5527, 39.7095) knots 0 0 0 1 2 2 2
  spline S84 degree 2 poles (-13.5527, 39.7095) (-15.2248, 39.7095) (-17.2604, 42.3357) (-17.2604, 44.5713) knots 0 0 0 1 2 2 2
  spline S85 degree 2 poles (-11.4535, 28.0593) (-14.1798, 28.0593) (-17.2968, 30.9673) (-17.2968, 33.4936) knots 0 0 0 1 2 2 2
  spline S86 degree 2 poles (-17.2968, 33.4936) (-17.2968, 36.029) (-14.1434, 38.9188) (-11.4535, 38.9188) knots 0 0 0 1 2 2 2
  spline S87 degree 2 poles (-11.4535, 38.9188) (-8.7545, 38.9188) (-5.6102, 36.029) (-5.6102, 33.4936) knots 0 0 0 1 2 2 2
  spline S88 degree 2 poles (-5.6102, 33.4936) (-5.6102, 30.9673) (-8.7363, 28.0593) (-11.4535, 28.0593) knots 0 0 0 1 2 2 2
  spline S89 degree 2 poles (-11.4535, 30.9673) (-10.4448, 30.9673) (-9.0362, 31.3762) (-8.5909, 31.7306) knots 0 0 0 1 2 2 2
  spline S90 degree 2 poles (-8.5909, 31.7306) (-8.1275, 32.085) (-7.7276, 32.9938) (-7.7276, 33.4845) knots 0 0 0 1 2 2 2
  spline S91 degree 2 poles (-7.7276, 33.4845) (-7.7276, 34.0025) (-8.1002, 34.8476) (-8.5728, 35.2384) knots 0 0 0 1 2 2 2
  spline S92 degree 2 poles (-8.5728, 35.2384) (-9.009, 35.5837) (-10.4539, 36.0108) (-11.4535, 36.0108) knots 0 0 0 1 2 2 2
  spline S93 degree 2 poles (-11.4535, 36.0108) (-12.4895, 36.0108) (-13.8526, 35.6019) (-14.3161, 35.2475) knots 0 0 0 1 2 2 2
  spline S94 degree 2 poles (-14.3161, 35.2475) (-14.7795, 34.8931) (-15.1794, 33.9752) (-15.1794, 33.4845) knots 0 0 0 1 2 2 2
  spline S95 degree 2 poles (-15.1794, 33.4845) (-15.1794, 32.9847) (-14.7523, 32.0578) (-14.2979, 31.7215) knots 0 0 0 1 2 2 2
  spline S96 degree 2 poles (-14.2979, 31.7215) (-13.8072, 31.358) (-12.5077, 30.9673) (-11.4535, 30.9673) knots 0 0 0 1 2 2 2
  spline S97 degree 2 poles (-11.4535, 16.1819) (-14.1798, 16.1819) (-17.2968, 19.0899) (-17.2968, 21.6162) knots 0 0 0 1 2 2 2
  spline S98 degree 2 poles (-17.2968, 21.6162) (-17.2968, 24.1516) (-14.1434, 27.0415) (-11.4535, 27.0415) knots 0 0 0 1 2 2 2
  spline S99 degree 2 poles (-11.4535, 27.0415) (-8.7545, 27.0415) (-5.6102, 24.1516) (-5.6102, 21.6162) knots 0 0 0 1 2 2 2
  spline S100 degree 2 poles (-5.6102, 21.6162) (-5.6102, 19.0899) (-8.7363, 16.1819) (-11.4535, 16.1819) knots 0 0 0 1 2 2 2
  spline S101 degree 2 poles (-11.4535, 19.0899) (-10.4448, 19.0899) (-9.0362, 19.4988) (-8.5909, 19.8532) knots 0 0 0 1 2 2 2
  spline S102 degree 2 poles (-8.5909, 19.8532) (-8.1275, 20.2076) (-7.7276, 21.1164) (-7.7276, 21.6071) knots 0 0 0 1 2 2 2
  spline S103 degree 2 poles (-7.7276, 21.6071) (-7.7276, 22.1251) (-8.1002, 22.9702) (-8.5728, 23.361) knots 0 0 0 1 2 2 2
  spline S104 degree 2 poles (-8.5728, 23.361) (-9.009, 23.7063) (-10.4539, 24.1334) (-11.4535, 24.1334) knots 0 0 0 1 2 2 2
  spline S105 degree 2 poles (-11.4535, 24.1334) (-12.4895, 24.1334) (-13.8526, 23.7245) (-14.3161, 23.3701) knots 0 0 0 1 2 2 2
  spline S106 degree 2 poles (-14.3161, 23.3701) (-14.7795, 23.0157) (-15.1794, 22.0978) (-15.1794, 21.6071) knots 0 0 0 1 2 2 2
  spline S107 degree 2 poles (-15.1794, 21.6071) (-15.1794, 21.1073) (-14.7523, 20.1804) (-14.2979, 19.8441) knots 0 0 0 1 2 2 2
  spline S108 degree 2 poles (-14.2979, 19.8441) (-13.8072, 19.4806) (-12.5077, 19.0899) (-11.4535, 19.0899) knots 0 0 0 1 2 2 2
  spline S109 degree 2 poles (-9.3816, 5.8857) (-10.1631, 5.8857) (-11.5807, 6.3855) (-12.0533, 6.849) knots 0 0 0 1 2 2 2
  spline S110 degree 2 poles (-12.0533, 6.849) (-12.3532, 7.1307) (-12.8439, 7.8213) (-13.0166, 8.2303) knots 0 0 0 1 2 2 2
  spline S111 degree 2 poles (-13.0166, 8.2303) (-13.1892, 8.6483) (-13.3892, 9.6207) (-13.3892, 10.2205) knots 0 0 0 1 2 2 2
  line L55 (-13.3892, 10.2205) -> (-13.3892, 11.6926)
  line L56 (-13.3892, 11.6926) -> (-17.0605, 11.6926)
  line L57 (-17.0605, 11.6926) -> (-17.0605, 14.5098)
  line L58 (-17.0605, 14.5098) -> (-5.8465, 14.5098)
  line L59 (-5.8465, 14.5098) -> (-5.8465, 10.1568)
  spline S112 degree 2 poles (-5.8465, 10.1568) (-5.8465, 9.1936) (-6.2009, 7.785) (-6.5826, 7.2125) knots 0 0 0 1 2 2 2
  spline S113 degree 2 poles (-6.5826, 7.2125) (-7.0097, 6.5764) (-8.4092, 5.8857) (-9.3816, 5.8857) knots 0 0 0 1 2 2 2
  spline S114 degree 2 poles (-9.4543, 8.7755) (-8.9726, 8.7755) (-8.2911, 9.2299) (-8.1638, 9.5389) knots 0 0 0 1 2 2 2
  spline S115 degree 2 poles (-8.1638, 9.5389) (-7.9912, 9.9387) (-7.9366, 10.6657) (-7.9366, 11.2928) knots 0 0 0 1 2 2 2
  line L60 (-7.9366, 11.2928) -> (-7.9366, 11.6926)
  line L61 (-7.9366, 11.6926) -> (-11.299, 11.6926)
  line L62 (-11.299, 11.6926) -> (-11.299, 11.4927)
  spline S116 degree 2 poles (-11.299, 11.4927) (-11.299, 11.1019) (-11.2808, 10.3931) (-11.2354, 10.1296) knots 0 0 0 1 2 2 2
  spline S117 degree 2 poles (-11.2354, 10.1296) (-11.1991, 9.9024) (-10.981, 9.4026) (-10.8446, 9.2663) knots 0 0 0 1 2 2 2
  spline S118 degree 2 poles (-10.8446, 9.2663) (-10.572, 8.9755) (-9.9632, 8.7755) (-9.4543, 8.7755) knots 0 0 0 1 2 2 2
  point P0 (0, 96.85)
  constraints: 2 other
extrude "Extrusion5" cut sketch "Skizze7" against normal blind 1
sketch "Skizze8" plane through (-45.65, -100.85, 24.3) normal (0, -1, 0) x (1, 0, 0)
  line L0 (70.15, 0) -> (70.15, -24.3) projected
  line L1 (44.9999, 0) -> (70.15, 0) projected
  line L2 (44.9999, 0) -> (44.9999, -14.1) projected
  line L3 (44.9999, -14.1) -> (24.9999, -14.1) projected
  line L4 (24.9999, -14.1) -> (24.9999, 0) projected
  line L5 (5.5, 0) -> (24.9999, 0) projected
  line L6 (-16.85, -24.3) -> (-16.85, 0) projected
  line L7 (-16.85, -24.3) -> (70.15, -24.3) projected
  line L8 (66.15, -20.3) -> (66.15, -4) construction
  line L9 (66.15, -4) -> (48.9999, -4) construction
  line L10 (48.9999, -4) -> (48.9999, -18.1) construction
  line L11 (48.9999, -18.1) -> (20.9999, -18.1) construction
  line L12 (20.9999, -18.1) -> (20.9999, -4) construction
  line L13 (20.9999, -4) -> (8.8917, -4) construction
  arc A0 (-8.8917, -4) -> (8.8917, -4) centre (0, 0) ccw construction
  line L14 (-8.8917, -4) -> (-12.85, -4) construction
  line L15 (-12.85, -4) -> (-12.85, -20.3) construction
  line L16 (-12.85, -20.3) -> (66.15, -20.3) construction
  arc A1 (-5.5, 0) -> (5.5, 0) centre (0, 0) ccw projected
  line L17 (-16.85, 0) -> (-5.5, 0) projected
  point P0 (45.65, -24.3)
  dimension "d42" = 4
  constraints: 18 end point, 8 coincident, 2 point on circle, 1 centre point, 6 other
  measures "d42" distance between parallel lines of L0 L8
hole "Bohrung2" at (20.5, -100.85, 4) at (20.5, -100.85, 20.3) at (3.3499, -100.85, 6.2) at (-24.6501, -100.85, 6.2) at (-24.6501, -100.85, 20.3) at (-58.5, -100.85, 20.3) at (3.3499, -100.85, 20.3) at (-58.5, -100.85, 4) direction (0, 1, 0) diameter 2.8 depth 12 tip angle 118
sketch "Skizze9" plane through (0, 0, 0) normal (0, 0, -1) x (-1, 0, 0)
  circle A0 centre (-15, -38.35) radius 1.35 projected
  circle A1 centre (43, -38.35) radius 1.35 projected
  circle A2 centre (43, -87.35) radius 1.35 projected
  circle A3 centre (-15, -87.35) radius 1.35 projected
  point P0 (0, 0)
hole "Bohrung3" at (15, -38.35, 0) at (-43, -38.35, 0) at (-43, -87.35, 0) at (15, -87.35, 0) direction (0, 0, 1) diameter 2.8 depth 12 tip angle 118
sketch "Skizze10" plane through (-66.5, -55.66, 16.6816) normal (-1, 0, 0) x (0, 0, 1)
  line L0 (-8.6816, 82.81) -> (7.6184, 82.81) projected
  line L1 (-8.6816, 82.81) -> (-8.6816, 81.56) projected
  line L2 (-8.6816, 81.56) -> (-16.6816, 81.56) projected
  line L3 (-16.6816, 81.56) -> (-16.6816, 61.06) projected
  line L4 (-16.6816, 61.06) -> (-8.6816, 61.06) projected
  line L5 (-8.6816, 61.06) -> (-8.6816, 58.56) projected
  line L6 (-8.6816, 58.56) -> (-16.6816, 58.56) projected
  line L7 (-16.6816, 58.56) -> (-16.6816, -41.19) projected
  line L8 (7.6184, -41.19) -> (-16.6816, -41.19) projected
  line L9 (7.6184, 0) -> (7.6184, -41.19) projected
  line L10 (-12.6816, -37.19) -> (-12.6816, 54.56) construction
  line L11 (-12.6816, 54.56) -> (-4.6816, 54.56) construction
  line L12 (-4.6816, 54.56) -> (-4.6816, 65.06) construction
  line L13 (-4.6816, 65.06) -> (-12.6816, 65.06) construction
  line L14 (-12.6816, 65.06) -> (-12.6816, 77.56) construction
  line L15 (-12.6816, 77.56) -> (-4.6816, 77.56) construction
  line L16 (-4.6816, 77.56) -> (-4.6816, 78.81) construction
  line L17 (-4.6816, 78.81) -> (3.6184, 78.81) construction
  line L18 (3.6184, 78.81) -> (3.6184, 23) construction
  line L19 (3.6184, 23) -> (-4, 23) construction
  line L20 (-4, 23) -> (-4, -4) construction
  line L21 (-4, -4) -> (3.6184, -4) construction
  line L22 (3.6184, -4) -> (3.6184, -37.19) construction
  line L23 (3.6184, -37.19) -> (-12.6816, -37.19) construction
  line L24 (7.6184, 0) -> (0, 0) projected
  line L25 (0, 0) -> (0, 19) projected
  line L26 (0, 19) -> (7.6184, 19) projected
  line L27 (7.6184, 82.81) -> (7.6184, 19) projected
  point P0 (-16.6816, 55.66)
  dimension "d57" = 4
  constraints: 28 end point, 6 coincident, 8 other
  measures "d57" distance between parallel lines of L8 L23
hole "Bohrung4" at (-66.5, -92.85, 20.3) at (-66.5, -92.85, 4) at (-66.5, -1.1, 4) at (-66.5, -32.66, 20.3) at (-66.5, 23.15, 20.3) at (-66.5, 21.9, 4) direction (1, 0, 0) diameter 2.8 depth 12 tip angle 118
sketch "Skizze11" plane through (28.5, -96.85, 0) normal (1, 0, 0) x (0, 0, -1)
  line L0 (-13.3892, 10.2205) -> (-13.3892, 11.6926) construction
  line L1 (-13.3892, 11.6926) -> (-17.0605, 11.6926) construction
  line L2 (-17.0605, 11.6926) -> (-17.0605, 14.5098) construction
  line L3 (-17.0605, 14.5098) -> (-5.8465, 14.5098) construction
  line L4 (-5.8465, 14.5098) -> (-5.8465, 10.1568) construction
  line L5 (-12.7621, 52.2684) -> (-17.0605, 49.1696) construction
  line L6 (-17.0605, 49.1696) -> (-17.0605, 52.2593) construction
  line L7 (-17.0605, 52.2593) -> (-14.6341, 53.8678) construction
  line L8 (-14.6341, 53.8678) -> (-17.0605, 55.5217) construction
  line L9 (-17.0605, 55.5217) -> (-17.0605, 58.5479) construction
  line L10 (-17.0605, 58.5479) -> (-12.8257, 55.4309) construction
  line L11 (-12.8257, 55.4309) -> (-8.6, 58.4934) construction
  line L12 (-8.6, 58.4934) -> (-8.6, 55.4036) construction
  line L13 (-8.6, 55.4036) -> (-10.981, 53.8224) construction
  line L14 (-10.981, 53.8224) -> (-8.6, 52.2321) construction
  line L15 (-8.6, 52.2321) -> (-8.6, 49.2059) construction
  line L16 (-8.6, 49.2059) -> (-12.7621, 52.2684) construction
  line L17 (-6.5917, 67.1901) -> (-8.391, 67.1901) construction
  line L18 (-8.391, 67.1901) -> (-8.391, 67.3083) construction
  line L19 (-14.516, 67.2992) -> (-14.516, 67.1901) construction
  line L20 (-14.516, 67.1901) -> (-16.2972, 67.1901) construction
  line L21 (-11.5989, 87.2735) -> (-17.0605, 87.2735) construction
  line L22 (-17.0605, 87.2735) -> (-17.0605, 88.6912) construction
  line L23 (-17.0605, 88.6912) -> (-12.2623, 88.6912) construction
  line L24 (-10.7719, 92.4625) -> (-17.0605, 92.4625) construction
  line L25 (-17.0605, 92.4625) -> (-17.0605, 93.8802) construction
  line L26 (-17.0605, 93.8802) -> (-8.6455, 93.8802) construction
  line L27 (-8.6455, 93.8802) -> (-8.6455, 92.4625) construction
  line L28 (-8.6455, 92.4625) -> (-9.5815, 92.4625) construction
  line L29 (-12.2259, 95.316) -> (-12.9984, 95.316) construction
  line L30 (-12.9984, 95.316) -> (-12.9984, 101.1411) construction
  line L31 (-14.9976, 95.5523) -> (-14.9976, 95.4705) construction
  line L32 (-14.9976, 95.4705) -> (-16.5425, 95.4705) construction
  line L33 (-16.6334, 109.1018) -> (-20.1594, 109.1018) construction
  line L34 (-20.1594, 109.1018) -> (-20.1594, 110.5194) construction
  line L35 (-20.1594, 110.5194) -> (-8.6455, 110.5194) construction
  line L36 (-8.6455, 110.5194) -> (-8.6455, 109.1018) construction
  line L37 (-8.6455, 109.1018) -> (-9.527, 109.1018) construction
  line L38 (-12.8439, 85.3106) -> (-5.8465, 85.3106) construction
  line L39 (-5.8465, 85.3106) -> (-5.8465, 83.8203) construction
  line L40 (-5.8465, 83.8203) -> (-12.8439, 83.8203) construction
  line L41 (-12.8802, 78.6858) -> (-5.8465, 78.6858) construction
  line L42 (-5.8465, 78.6858) -> (-5.8465, 77.1955) construction
  line L43 (-5.8465, 77.1955) -> (-12.8439, 77.1955) construction
  line L44 (-15.761, 59.2022) -> (-17.0605, 59.2022) construction
  line L45 (-17.0605, 59.2022) -> (-17.0605, 66.1178) construction
  line L46 (-17.0605, 66.1178) -> (-15.4702, 66.1178) construction
  line L47 (-7.8821, 65.7997) -> (-7.8821, 65.8815) construction
  line L48 (-7.8821, 65.8815) -> (-6.2827, 65.8815) construction
  line L49 (-15.761, 64.7092) -> (-15.761, 59.2022) construction
  line L50 (-16.3971, 48.6425) -> (-13.7254, 48.6425) construction
  line L51 (-13.7254, 48.6425) -> (-13.7254, 48.388) construction
  line L52 (-6.4008, 40.1547) -> (-8.9635, 40.1547) construction
  line L53 (-8.9635, 40.1547) -> (-8.9635, 40.4001) construction
  line L54 (-24.3, 124) -> (0, 124) construction
  line L55 (-24.3, 0) -> (-24.3, 124) construction
  line L56 (0, 0) -> (-24.3, 0) construction
  line L57 (0, 0) -> (0, 124) construction
  line L58 (-20.3, 4) -> (-20.3, 120) construction
  line L59 (-20.3, 120) -> (-4, 120) construction
  line L60 (-4, 120) -> (-4, 4) construction
  line L61 (-4, 4) -> (-20.3, 4) construction
  point P0 (0, 96.85)
  dimension "d65" = 4
  constraints: 8 end point, 4 coincident, 89 other
  measures "d65" distance between parallel lines of L56 L61
hole "Bohrung5" at (28.5, -92.85, 4) at (28.5, -92.85, 20.3) at (28.5, 23.15, 4) at (28.5, 23.15, 20.3) direction (-1, 0, 0) diameter 2.8 depth 12 tip angle 118
fillet "Rundung1" radius 2 1 edges at (-66.5, -46.16, 16.6816)
sketch "Skizze12" plane through (-66.5, 31.15, 10.2) normal (0, 0, 1) x (1, 0, 0)
  line L0 (56.7131, -74.6503) -> (56.7131, -86.81) projected
  line L1 (56.7131, -86.81) -> (51.6692, -86.81) projected
  line L2 (51.6692, -88.26) -> (51.6692, -86.81) projected
  line L3 (44.3499, -88.26) -> (51.6692, -88.26) projected
  line L4 (44.3499, -90.06) -> (44.3499, -88.26) projected
  line L5 (41.3499, -90.06) -> (44.3499, -90.06) projected
  line L6 (41.3499, -122.56) -> (41.3499, -90.06) projected
  line L7 (45.8499, -122.56) -> (41.3499, -122.56) projected
  line L8 (45.8499, -132) -> (45.8499, -122.56) projected
  line L9 (65.8499, -132) -> (45.8499, -132) projected
  line L10 (65.8499, -122.56) -> (65.8499, -132) projected
  line L11 (70.3499, -122.56) -> (65.8499, -122.56) projected
  line L12 (70.3499, -90.06) -> (70.3499, -122.56) projected
  line L13 (67.3499, -90.06) -> (70.3499, -90.06) projected
  line L14 (67.3499, -88.26) -> (67.3499, -90.06) projected
  line L15 (60.0306, -88.26) -> (67.3499, -88.26) projected
  line L16 (60.0306, -74.6503) -> (60.0306, -88.26) projected
  line L17 (56.7131, -74.6503) -> (60.0306, -74.6503) projected
  line L18 (70.3499, -90.06) -> (70.3499, -122.56) projected
  line L19 (41.3499, -122.56) -> (70.3499, -122.56)
  line L20 (70.3499, -122.56) -> (70.3499, -115.56)
  line L21 (70.3499, -115.56) -> (41.3499, -115.56)
  line L22 (41.3499, -115.56) -> (41.3499, -122.56)
  point P0 (66.5, -31.15)
  dimension "d77" = 7
  constraints: 8 end point, 2 parallel, 1 horizontal, 1 perpendicular, 1 point on line
  measures "d77" distance of L20.end L19.end
extrude "Extrusion6" cut sketch "Skizze12" against normal through all contours L12 L11 L19 L7 L6 L21